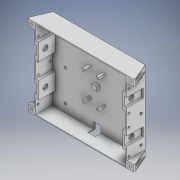
# Autodesk Inventor part: IPC Rear Panel v2
Saved by Autodesk Inventor 2022 (Build 260153000, 153)
## iProperties
Created: 2021-12-31
Part Number: IPC Rear Panel v2
Material: Generic
Document SubType Name: Modeling
Designer: solor
Density: 1 g/cm^3
Appearance: Default
Author: solor
Autodesk Inventor part; units mm, degrees
ref_plane "YZ Plane" through (0, 0, 0) normal (1, 0, 0) x (0, 1, 0)
ref_plane "XZ Plane" through (0, 0, 0) normal (0, 1, 0) x (-1, 0, 0)
sketch "Sketch1" plane through (0, 0, 0) normal (0, 0, 1) x (1, 0, 0)
  line L0 (0, 106) -> (0, 97)
  line L1 (0, 97) -> (9, 97)
  line L2 (9, 9) -> (0, 9)
  line L3 (0, 9) -> (0, 0)
  line L4 (138.8502, 0) -> (138.8502, 9)
  line L5 (138.8502, 9) -> (129.8502, 9)
  line L6 (129.8502, 97) -> (138.8502, 97)
  line L7 (138.8502, 97) -> (138.8502, 106)
  circle A0 centre (134.3502, 101.5) radius 1.65
  circle A1 centre (134.3502, 4.5) radius 1.65
  circle A2 centre (4.5, 4.5) radius 1.65
  circle A3 centre (4.5, 101.5) radius 1.65
  line L8 (9, 106) -> (9, 0)
  line L9 (129.8502, 0) -> (129.8502, 106)
  line L10 (0, 106) -> (9, 106)
  line L11 (9, 106) -> (129.8502, 106)
  line L12 (129.8502, 106) -> (138.8502, 106)
  line L13 (138.8502, 0) -> (129.8502, 0)
  line L14 (129.8502, 0) -> (9, 0)
  line L15 (9, 0) -> (0, 0)
  line L16 (10.3351, 1.335) -> (128.5151, 1.335)
  line L17 (128.5151, 1.335) -> (128.5151, 104.665)
  line L18 (128.5151, 104.665) -> (10.3351, 104.665)
  line L19 (10.3351, 104.665) -> (10.3351, 1.335)
  line L20 (10.3351, 1.335) -> (128.5151, 104.665) construction
  line L21 (128.5151, 1.335) -> (10.3351, 104.665) construction
  point P0 (0, 0)
  point P1 (69.4251, 53)
  dimension "d0" = 118.18
  dimension "d1" = 103.33
  constraints: 44 end point, 4 centre point, 4 collinear, 4 point on line, 3 parallel, 2 horizontal, 2 midpoint, 1 perpendicular
  measures "d0" distance of L18.end L17.end
  measures "d1" distance of L17.end L16.end
sketch "Sketch2" plane through (0, 0, 0) normal (0, 0, 1) x (1, 0, 0)
  line L0 (9, 46.5) -> (9, 9)
  line L1 (0, 46.5) -> (9, 46.5)
  line L2 (0, 59.5) -> (0, 46.5)
  line L3 (9, 59.5) -> (0, 59.5)
  line L4 (9, 88) -> (9, 59.5)
  line L5 (9, 97) -> (9, 88)
  line L6 (9, 97) -> (0, 97)
  line L7 (0, 97) -> (0, 106)
  line L8 (117.3502, 0) -> (3.5, 0)
  line L9 (117.3502, 0) -> (129.8502, 0)
  line L10 (138.8502, 106) -> (138.8502, 97)
  line L11 (138.8502, 97) -> (129.8502, 97)
  line L12 (129.8502, 88) -> (129.8502, 97)
  line L13 (129.8502, 59.5) -> (129.8502, 88)
  line L14 (138.8502, 59.5) -> (129.8502, 59.5)
  line L15 (138.8502, 46.5) -> (138.8502, 59.5)
  line L16 (129.8502, 46.5) -> (138.8502, 46.5)
  line L17 (129.8502, 9) -> (129.8502, 46.5)
  line L18 (129.8502, 9) -> (138.8502, 9)
  line L19 (138.8502, 9) -> (138.8502, 0)
  line L20 (138.8502, 0) -> (126.3502, 0)
  line L21 (12.5, 0) -> (126.3502, 0)
  line L22 (12.5, 0) -> (0, 0)
  line L23 (0, 0) -> (0, 9)
  line L24 (0, 9) -> (9, 9)
  circle A0 centre (4.5, 4.5) radius 1.65
  circle A1 centre (134.3502, 4.5) radius 1.65
  circle A2 centre (134.3502, 101.5) radius 1.65
  circle A3 centre (4.5, 101.5) radius 1.65
  constraints: 50 end point, 4 centre point
extrude "Extrusion1" add sketch "Sketch1" along normal blind 24 contours L11 L9 L14 L8
extrude "Extrusion2" add sketch "Sketch1" along normal blind 2.56 contours L19 L18 L17 L16
sketch "Sketch3" plane through (0, 0, 24) normal (0, 0, 1) x (1, 0, 0)
  line L0 (138.8502, 97) -> (129.8502, 97) projected
  line L1 (138.8502, 106) -> (138.8502, 97) projected
  line L2 (129.8502, 106) -> (138.8502, 106) projected
  circle A0 centre (134.3502, 101.5) radius 1.65 projected
  line L3 (129.8502, 0) -> (129.8502, 106) projected
  line L4 (129.8502, 9) -> (138.8502, 9) projected
  line L5 (138.8502, 9) -> (138.8502, 0) projected
  line L6 (138.8502, 0) -> (126.3502, 0) projected
  circle A1 centre (134.3502, 4.5) radius 1.65 projected
  line L7 (12.5, 0) -> (0, 0) projected
  line L8 (0, 0) -> (0, 9) projected
  line L9 (0, 9) -> (9, 9) projected
  circle A2 centre (4.5, 4.5) radius 1.65 projected
  line L10 (9, 97) -> (0, 97) projected
  line L11 (0, 97) -> (0, 106) projected
  line L12 (0, 106) -> (9, 106) projected
  circle A3 centre (4.5, 101.5) radius 1.65 projected
  line L13 (9, 106) -> (9, 0) projected
extrude "Extrusion3" add sketch "Sketch3" against normal blind 2.56
sketch "Sketch4" plane through (9, 0, 0) normal (0, -1, 0) x (1, 0, 0)
  line L0 (0, 21.44) -> (-9, 21.44) projected
  line L1 (0, 0) -> (0, 21.44) projected
  line L2 (-9, 21.44) -> (0, 0)
  line L3 (0, 0) -> (0, 21.44)
  line L4 (0, 21.44) -> (-9, 21.44)
  line L5 (120.8502, 0) -> (120.8502, 21.44) projected
  line L6 (129.8502, 21.44) -> (120.8502, 21.44) projected
  line L7 (120.8502, 21.44) -> (129.8502, 21.44)
  line L8 (129.8502, 21.44) -> (120.8502, 0)
  line L9 (120.8502, 0) -> (120.8502, 21.44)
  point P0 (-9, 0)
  constraints: 12 end point, 2 perpendicular, 1 collinear, 1 horizontal
extrude "Extrusion4" add sketch "Sketch4" against normal blind 106
sketch "Sketch5" plane through (138.8502, 97, 24) normal (1, 0, 0) x (0, 0, -1)
  line L0 (2.56, 0) -> (2.56, -88) projected
  line L1 (2.56, -88) -> (25.0861, -88)
  line L2 (24, -97) -> (24, 9) projected
  line L3 (25.0861, -88) -> (25.0861, 0)
  line L4 (25.0861, 0) -> (-1.4553, 0)
  line L5 (-1.4553, 0) -> (-1.4553, -88)
  line L6 (2.56, -88) -> (0, -88) projected
  line L7 (-1.4553, -88) -> (2.56, -88)
  line L8 (2.56, -97) -> (2.56, -88) projected
  line L9 (2.56, -88) -> (2.56, -89.3)
  line L10 (2.56, -89.3) -> (24, -89.3)
  line L11 (24, -89.3) -> (24, -95.7)
  line L12 (24, -95.7) -> (2.56, -95.7)
  line L13 (2.56, -95.7) -> (2.56, -89.3)
  line L14 (2.56, 9) -> (2.56, 0) projected
  line L15 (2.56, 0) -> (2.56, 1.3)
  line L16 (2.56, 1.3) -> (24, 1.3)
  line L17 (24, 1.3) -> (24, 7.7)
  line L18 (24, 7.7) -> (2.56, 7.7)
  line L19 (2.56, 7.7) -> (2.56, 1.3)
  point P0 (2.56, 7.7)
  point P1 (24, 0)
  point P2 (24, -88)
  dimension "d10" = 1.3
  dimension "d11" = 6.4
  dimension "d12" = 1.3
  dimension "d13" = 6.4
  constraints: 30 end point, 10 perpendicular, 9 point on line, 1 collinear
  measures "d10" distance of L0.end L9.end
  measures "d11" distance of L10.end L11.end
  measures "d12" distance of L0.start L15.end
  measures "d13" distance of L16.end L17.end
extrude "Extrusion5" cut sketch "Sketch5" against normal blind 9 contours L4 L2 L1 L0 | L14 L18 L2 L16 | L10 L2 L12 L8
sketch "Sketch6" plane through (0, 0, 24) normal (-1, 0, 0) x (0, 0, 1)
  line L0 (-24, 1.3) -> (-24, 7.7) projected
  line L1 (-2.56, 7.7) -> (-24, 7.7) projected
  line L2 (-2.56, 1.3) -> (-2.56, 7.7) projected
  line L3 (-24, 1.3) -> (-2.56, 1.3) projected
  line L4 (-24, 97) -> (0, 97) projected
  line L5 (0, 9) -> (0, 97) projected
  line L6 (0, 9) -> (-24, 9) projected
  line L7 (-24, 9) -> (-24, 97) projected
  line L8 (-2.56, 98.3) -> (-2.56, 104.7) projected
  line L9 (-24, 98.3) -> (-2.56, 98.3) projected
  line L10 (-24, 98.3) -> (-24, 104.7) projected
  line L11 (-2.56, 104.7) -> (-24, 104.7) projected
  point P0 (-24, 0)
extrude "Extrusion6" cut sketch "Sketch6" against normal blind 9
ref_plane "Work Plane1" through (0, 0, 37.6398) normal (0, 0, 1) x (1, 0, 0)
sketch "Sketch7" plane through (0, 0, 37.6398) normal (0, 0, 1) x (1, 0, 0)
  line L0 (0, 59.5) -> (0, 46.5) projected
  line L1 (9, 59.5) -> (0, 59.5) projected
  line L2 (0, 46.5) -> (9, 46.5) projected
  line L3 (9, 97) -> (9, 9) projected
  line L4 (138.8502, 46.5) -> (138.8502, 59.5) projected
  line L5 (129.8502, 46.5) -> (138.8502, 46.5) projected
  line L6 (138.8502, 59.5) -> (129.8502, 59.5) projected
  line L7 (129.8502, 9) -> (129.8502, 97) projected
  point P0 (0, 0)
sketch "Sketch8" plane through (9, 9, 24) normal (-1, 0, 0) x (0, 0, 1)
  line L0 (32.712, 88) -> (32.712, 50.5) construction
  line L1 (17.6212, 69.25) -> (-0.9488, 69.25) construction
  line L2 (0, -16.3005) -> (-7, -16.3005) construction
  line L3 (13.6398, 37.5) -> (13.6398, 50.5) construction
  line L4 (13.6398, 44) -> (-26.4859, 44) construction
  line L5 (-34.861, 44) -> (-34.861, 88) construction
  circle A0 centre (-7, 66) radius 21.6937
  circle A1 centre (-7, 66) radius 5.75
  point P0 (-24, -9)
  dimension "d21" = 18.57
  dimension "d23" = 7
  dimension "d24" = 11.5
  constraints: 10 end point, 3 horizontal, 2 centre point, 2 vertical, 1 coincident, 1 midpoint
  measures "d21" distance of L1.start L1.end
  measures "d23" distance of L2.start L2.end
  measures "d24" diameter of A1
sketch "Sketch9" plane through (0, 0, 24) normal (0, 0, 1) x (1, 0, 0)
  line L0 (14.2, 69.25) -> (14.2, 80.75)
  line L1 (14.2, 80.75) -> (9, 80.75)
  line L2 (9, 86.2) -> (16.78, 86.2)
  line L3 (16.78, 86.2) -> (16.78, 63.8)
  line L4 (16.78, 63.8) -> (9, 63.8)
  line L5 (9, 63.8) -> (9, 69.25)
  line L6 (9, 80.75) -> (9, 86.2)
  line L7 (9, 97) -> (9, 9) projected
  line L8 (9, 69.25) -> (14.2, 69.25)
  point P0 (0, 0)
  dimension "d29" = 7.78
  dimension "d30" = 22.4
  constraints: 16 end point, 2 perpendicular, 1 collinear, 1 parallel, 1 vertical
  measures "d29" distance of L2.start L2.end
  measures "d30" distance of L2.end L3.end
extrude "Extrusion8" add sketch "Sketch9" against normal blind 24 contours L0 L1 L6 L2 L3 L4 L5 L8
sketch "Sketch10" plane through (0, 0, 24) normal (0, 0, 1) x (1, 0, 0)
  line L0 (16.78, 63.8) -> (16.78, 86.2) projected
  line L1 (14.2, 69.25) -> (10.3351, 69.25) projected
  line L2 (14.2, 80.75) -> (14.2, 69.25) projected
  line L3 (10.3351, 69.25) -> (14.2, 69.25) projected
  line L4 (14.2, 69.25) -> (14.2, 80.75) projected
  line L5 (14.2, 80.75) -> (10.3351, 80.75) projected
  line L6 (10.3351, 69.25) -> (10.3351, 80.75) projected
  line L7 (10.3351, 104.665) -> (128.5151, 104.665) projected
  line L8 (69.4251, 104.665) -> (69.4251, 1.335)
  line L9 (128.5151, 1.335) -> (10.3351, 1.335) projected
  line L10 (9, 53) -> (129.7844, 53)
  line L11 (16.78, 86.2) -> (10.3351, 86.2) projected
  line L12 (10.3351, 69.25) -> (10.3351, 80.75) projected
  line L13 (10.3351, 80.75) -> (9, 80.75)
  line L14 (9, 80.75) -> (9, 69.25)
  line L15 (9, 69.25) -> (10.3351, 69.25)
  line L16 (10.3351, 80.75) -> (14.2, 80.75) projected
  line L17 (10.3351, 80.75) -> (10.3351, 69.25)
  line L18 (16.78, 63.8) -> (10.3351, 63.8) projected
  line L19 (10.3351, 63.8) -> (10.3351, 69.25)
  line L20 (10.3351, 86.2) -> (10.3351, 80.75)
  line L21 (122.0702, 63.8) -> (122.0702, 86.2)
  line L22 (124.6502, 69.25) -> (128.5151, 69.25)
  line L23 (124.6502, 80.75) -> (124.6502, 69.25)
  line L24 (128.5151, 69.25) -> (124.6502, 69.25)
  line L25 (124.6502, 69.25) -> (124.6502, 80.75)
  line L26 (124.6502, 80.75) -> (128.5151, 80.75)
  line L27 (128.5151, 69.25) -> (128.5151, 80.75)
  line L28 (122.0702, 86.2) -> (128.5151, 86.2)
  line L29 (128.5151, 69.25) -> (128.5151, 80.75)
  line L30 (128.5151, 80.75) -> (129.8502, 80.75)
  line L31 (129.8502, 80.75) -> (129.8502, 69.25)
  line L32 (129.8502, 69.25) -> (128.5151, 69.25)
  line L33 (128.5151, 80.75) -> (124.6502, 80.75)
  line L34 (128.5151, 80.75) -> (128.5151, 69.25)
  line L35 (122.0702, 63.8) -> (128.5151, 63.8)
  line L36 (128.5151, 63.8) -> (128.5151, 69.25)
  line L37 (128.5151, 86.2) -> (128.5151, 80.75)
  line L38 (16.78, 42.2) -> (16.78, 19.8)
  line L39 (14.2, 36.75) -> (10.3351, 36.75)
  line L40 (14.2, 25.25) -> (14.2, 36.75)
  line L41 (10.3351, 36.75) -> (14.2, 36.75)
  line L42 (14.2, 36.75) -> (14.2, 25.25)
  line L43 (14.2, 25.25) -> (10.3351, 25.25)
  line L44 (10.3351, 36.75) -> (10.3351, 25.25)
  line L45 (16.78, 19.8) -> (10.3351, 19.8)
  line L46 (10.3351, 36.75) -> (10.3351, 25.25)
  line L47 (10.3351, 25.25) -> (9, 25.25)
  line L48 (9, 25.25) -> (9, 36.75)
  line L49 (9, 36.75) -> (10.3351, 36.75)
  line L50 (10.3351, 25.25) -> (14.2, 25.25)
  line L51 (10.3351, 25.25) -> (10.3351, 36.75)
  line L52 (16.78, 42.2) -> (10.3351, 42.2)
  line L53 (10.3351, 42.2) -> (10.3351, 36.75)
  line L54 (10.3351, 19.8) -> (10.3351, 25.25)
  line L55 (122.0702, 42.2) -> (128.5151, 42.2)
  line L56 (124.6502, 36.75) -> (128.5151, 36.75)
  line L57 (128.5151, 36.75) -> (124.6502, 36.75)
  line L58 (128.5151, 42.2) -> (128.5151, 36.75)
  line L59 (129.8502, 36.75) -> (128.5151, 36.75)
  line L60 (124.6502, 25.25) -> (124.6502, 36.75)
  line L61 (124.6502, 36.75) -> (124.6502, 25.25)
  line L62 (122.0702, 42.2) -> (122.0702, 19.8)
  line L63 (128.5151, 25.25) -> (124.6502, 25.25)
  line L64 (128.5151, 36.75) -> (128.5151, 25.25)
  line L65 (128.5151, 25.25) -> (128.5151, 36.75)
  line L66 (128.5151, 36.75) -> (128.5151, 25.25)
  line L67 (124.6502, 25.25) -> (128.5151, 25.25)
  line L68 (122.0702, 19.8) -> (128.5151, 19.8)
  line L69 (129.8502, 25.25) -> (129.8502, 36.75)
  line L70 (128.5151, 19.8) -> (128.5151, 25.25)
  line L71 (128.5151, 25.25) -> (129.8502, 25.25)
  point P0 (0, 0)
  constraints: 118 end point, 39 symmetric about line, 3 perpendicular, 2 horizontal, 2 midpoint, 1 collinear
extrude "Extrusion9" cut sketch "Sketch10" against normal blind 21.44 contours L15 L14 L13 L6 | L27 L30 L31 L32 | L44 L47 L48 L49 | L59 L69 L71 L64
extrude "Extrusion10" add sketch "Sketch10" against normal blind 21.44 contours L21 L28 L37 L26 L23 L22 L36 L35 | L38 L45 L54 L43 L40 L39 L53 L52 | L55 L58 L56 L60 L63 L70 L68 L62
sketch "Sketch11" plane through (9, 9, 0) normal (-1, 0, 0) x (0, 0, 1)
  line L0 (2.56, 33.2) -> (2.56, 10.8) projected
  circle A0 centre (17, 66) radius 21.6937 projected
  line L1 (24, 27.75) -> (2.56, 27.75) projected
  circle A1 centre (17, 22) radius 21.6937
  circle A2 centre (17, 66) radius 3.525
  circle A3 centre (17, 22) radius 3.525
  line L2 (9.65, 22) -> (9.65, 23.5)
  line L3 (9.65, 23.5) -> (7.65, 23.5)
  line L4 (7.65, 23.5) -> (7.65, 20.5)
  line L5 (7.65, 20.5) -> (9.65, 20.5)
  line L6 (9.65, 20.5) -> (9.65, 22)
  line L7 (37.6398, 37.5) -> (37.6398, 50.5) projected
  line L8 (37.6398, 44) -> (44.1108, 44)
  line L9 (9.65, 66) -> (9.65, 64.5)
  line L10 (9.65, 64.5) -> (7.65, 64.5)
  line L11 (7.65, 64.5) -> (7.65, 67.5)
  line L12 (7.65, 67.5) -> (9.65, 67.5)
  line L13 (9.65, 67.5) -> (9.65, 66)
  line L14 (17, 31.5257) -> (17, 36.9305)
  line L15 (24.35, 22) -> (24.35, 23.5)
  line L16 (24.35, 23.5) -> (26.35, 23.5)
  line L17 (26.35, 23.5) -> (26.35, 20.5)
  line L18 (26.35, 20.5) -> (24.35, 20.5)
  line L19 (24.35, 20.5) -> (24.35, 22)
  line L20 (24.35, 64.5) -> (26.35, 64.5)
  line L21 (24.35, 66) -> (24.35, 64.5)
  line L22 (24.35, 67.5) -> (24.35, 66)
  line L23 (26.35, 64.5) -> (26.35, 67.5)
  line L24 (26.35, 67.5) -> (24.35, 67.5)
  point P0 (0, -9)
  point P1 (2.56, 22)
  dimension "d37" = 7.05
  dimension "d38" = 7.05
  constraints: 44 end point, 15 symmetric about line, 4 perpendicular, 4 point on line, 3 centre point, 2 coincident, 2 midpoint, 1 horizontal, 1 vertical
  measures "d37" diameter of A2
  measures "d38" diameter of A3
extrude "Extrusion11" cut sketch "Sketch11" against normal blind 146.835 contours A2 | A3 | L6 L5 L4 L3 L2 | L9 L10 L11 L12 L13
sketch "Sketch12" plane through (0, 0, 24) normal (0, -1, 0) x (1, 0, 0)
  line L0 (66.4498, -24.1403) -> (72.4005, -24.1403)
  line L1 (72.4005, -24.1403) -> (72.4005, -17.0714)
  line L2 (72.4005, -17.0714) -> (66.4498, -17.0714)
  line L3 (66.4498, -17.0714) -> (66.4498, -24.1403)
  line L4 (66.4498, -24.1403) -> (72.4005, -17.0714) construction
  line L5 (72.4005, -24.1403) -> (66.4498, -17.0714) construction
  point P0 (0, -24)
  point P1 (69.4251, -20.6058)
  constraints: 12 end point, 2 midpoint, 2 parallel, 1 horizontal, 1 perpendicular
extrude "Extrusion12" cut sketch "Sketch12" against normal blind 5.5475
sketch "Sketch13" plane through (0, 0, 2.56) normal (0, 0, 1) x (1, 0, 0)
  line L0 (66.4498, 1.335) -> (66.4498, 5.5475) projected
  line L1 (66.4498, 5.5475) -> (72.4005, 5.5475) projected
  line L2 (72.4005, 5.5475) -> (72.4005, 1.335) projected
  line L3 (128.5151, 1.335) -> (72.4005, 1.335) projected
  line L4 (128.5151, 19.8) -> (128.5151, 1.335) projected
  line L5 (128.5151, 19.8) -> (122.0702, 19.8) projected
  line L6 (122.0702, 19.8) -> (122.0702, 42.2) projected
  line L7 (122.0702, 42.2) -> (128.5151, 42.2) projected
  line L8 (128.5151, 63.8) -> (128.5151, 42.2) projected
  line L9 (128.5151, 63.8) -> (122.0702, 63.8) projected
  line L10 (122.0702, 63.8) -> (122.0702, 86.2) projected
  line L11 (122.0702, 86.2) -> (128.5151, 86.2) projected
  line L12 (128.5151, 104.665) -> (128.5151, 86.2) projected
  line L13 (10.3351, 104.665) -> (128.5151, 104.665) projected
  line L14 (10.3351, 86.2) -> (10.3351, 104.665) projected
  line L15 (10.3351, 86.2) -> (16.78, 86.2) projected
  line L16 (16.78, 86.2) -> (16.78, 63.8) projected
  line L17 (16.78, 63.8) -> (10.3351, 63.8) projected
  line L18 (10.3351, 42.2) -> (10.3351, 63.8) projected
  line L19 (10.3351, 42.2) -> (16.78, 42.2) projected
  line L20 (16.78, 42.2) -> (16.78, 19.8) projected
  line L21 (16.78, 19.8) -> (10.3351, 19.8) projected
  line L22 (10.3351, 1.335) -> (10.3351, 19.8) projected
  line L23 (66.4498, 1.335) -> (10.3351, 1.335) projected
  line L24 (61.1838, 36.7005) -> (78.4251, 70.8) construction
  line L25 (78.4251, 35.2) -> (60.4251, 70.8) construction
  line L26 (61.9251, 33.5865) -> (61.9251, 35.2)
  line L27 (69.4251, 57.7505) -> (69.4251, 50.8052)
  line L28 (66.4498, 53) -> (71.4698, 53)
  line L29 (61.9251, 72.4135) -> (61.9251, 70.8)
  line L30 (60.4251, 69.2995) -> (58.8116, 69.2995)
  line L31 (76.9251, 33.5865) -> (76.9251, 35.2)
  line L32 (78.4251, 36.7005) -> (80.0387, 36.7005)
  line L33 (76.9251, 72.4135) -> (76.9251, 70.8)
  line L34 (78.4251, 69.2995) -> (80.0387, 69.2995)
  line L35 (60.4251, 36.7005) -> (58.8116, 36.7005)
  line L36 (60.4251, 70.8) -> (60.4251, 69.2995)
  line L37 (60.4251, 36.7005) -> (60.4251, 35.2)
  line L38 (58.8116, 33.5865) -> (58.8116, 36.7005)
  line L39 (58.8116, 69.2995) -> (58.8116, 72.4135)
  line L40 (58.8116, 72.4135) -> (61.9251, 72.4135)
  line L41 (76.9251, 72.4135) -> (80.0387, 72.4135)
  line L42 (78.4251, 70.8) -> (76.9251, 70.8)
  line L43 (61.9251, 70.8) -> (60.4251, 70.8)
  line L44 (78.4251, 35.2) -> (78.4251, 36.7005)
  line L45 (78.4251, 69.2995) -> (78.4251, 70.8)
  line L46 (80.0387, 72.4135) -> (80.0387, 69.2995)
  line L47 (80.0387, 36.7005) -> (80.0387, 33.5865)
  line L48 (60.4251, 35.2) -> (61.9251, 35.2)
  line L49 (76.9251, 35.2) -> (78.4251, 35.2)
  line L50 (80.0387, 33.5865) -> (76.9251, 33.5865)
  line L51 (61.9251, 33.5865) -> (58.8116, 33.5865)
  line L52 (66.0452, 50.056) -> (72.805, 50.056)
  line L53 (72.805, 50.056) -> (72.805, 55.944)
  line L54 (72.805, 55.944) -> (66.0452, 55.944)
  line L55 (66.0452, 55.944) -> (66.0452, 50.056)
  line L56 (66.0452, 50.056) -> (72.805, 55.944) construction
  line L57 (72.805, 50.056) -> (66.0452, 55.944) construction
  point P0 (0, 0)
  point P1 (69.4251, 53)
  point P2 (61.9251, 32.5085)
  point P3 (57.4575, 36.7005)
  point P4 (61.9251, 73.4915)
  point P5 (61.9251, 69.2995)
  point P6 (57.4575, 69.2995)
  point P7 (76.9251, 32.5085)
  point P8 (81.3927, 36.7005)
  point P9 (76.9251, 73.4915)
  point P10 (76.9251, 69.2995)
  point P11 (81.3927, 69.2995)
  dimension "d47" = 18
  dimension "d48" = 35.6
  constraints: 68 end point, 18 parallel, 13 perpendicular, 7 symmetric about line, 4 horizontal, 3 midpoint, 1 point on line, 1 vertical
  measures "d47" distance of L25.end L24.end
  measures "d48" distance of L24.end L25.start
extrude "Extrusion13" add sketch "Sketch13" along normal blind 8.7225 contours L51 L38 L35 L37 L48 L26 | L29 L43 L36 L30 L39 L40 | L31 L49 L44 L32 L47 L50 | L41 L46 L34 L45 L42 L33
extrude "Extrusion14" add sketch "Sketch13" along normal blind 4 contours L55 L54 L53 L52
sketch "Sketch14" plane through (0, 0, 2.56) normal (0, 0, 1) x (1, 0, 0)
  line L0 (66.0452, 55.944) -> (66.0452, 50.056) projected
  line L1 (66.0452, 50.056) -> (72.805, 50.056) projected
  line L2 (72.805, 50.056) -> (72.805, 55.944) projected
  line L3 (72.805, 55.944) -> (66.0452, 55.944) projected
  line L4 (66.0452, 55.944) -> (72.805, 55.944) projected
  line L5 (72.805, 55.944) -> (72.805, 50.056) projected
  line L6 (72.805, 50.056) -> (66.0452, 50.056) projected
  line L7 (66.0452, 50.056) -> (66.0452, 55.944) projected
  line L8 (78.4251, 69.2995) -> (78.4251, 70.8) projected
  line L9 (78.4251, 70.8) -> (76.9251, 70.8) projected
  line L10 (76.9251, 70.8) -> (76.9251, 72.4135) projected
  line L11 (76.9251, 72.4135) -> (80.0387, 72.4135) projected
  line L12 (80.0387, 72.4135) -> (80.0387, 69.2995) projected
  line L13 (80.0387, 69.2995) -> (78.4251, 69.2995) projected
  line L14 (80.0387, 33.5865) -> (76.9251, 33.5865) projected
  line L15 (76.9251, 33.5865) -> (76.9251, 35.2) projected
  line L16 (76.9251, 35.2) -> (78.4251, 35.2) projected
  line L17 (78.4251, 35.2) -> (78.4251, 36.7005) projected
  line L18 (78.4251, 36.7005) -> (80.0387, 36.7005) projected
  line L19 (80.0387, 36.7005) -> (80.0387, 33.5865) projected
  line L20 (58.8116, 72.4135) -> (61.9251, 72.4135) projected
  line L21 (61.9251, 72.4135) -> (61.9251, 70.8) projected
  line L22 (61.9251, 70.8) -> (60.4251, 70.8) projected
  line L23 (60.4251, 70.8) -> (60.4251, 69.2995) projected
  line L24 (60.4251, 69.2995) -> (58.8116, 69.2995) projected
  line L25 (58.8116, 69.2995) -> (58.8116, 72.4135) projected
  line L26 (61.9251, 33.5865) -> (58.8116, 33.5865) projected
  line L27 (58.8116, 33.5865) -> (58.8116, 36.7005) projected
  line L28 (58.8116, 36.7005) -> (60.4251, 36.7005) projected
  line L29 (60.4251, 36.7005) -> (60.4251, 35.2) projected
  line L30 (60.4251, 35.2) -> (61.9251, 35.2) projected
  line L31 (61.9251, 35.2) -> (61.9251, 33.5865) projected
  line L32 (66.4498, 1.335) -> (66.4498, 5.5475) projected
  line L33 (66.4498, 5.5475) -> (72.4005, 5.5475) projected
  line L34 (72.4005, 5.5475) -> (72.4005, 1.335) projected
  line L35 (128.5151, 1.335) -> (72.4005, 1.335) projected
  line L36 (128.5151, 19.8) -> (128.5151, 1.335) projected
  line L37 (128.5151, 19.8) -> (122.0702, 19.8) projected
  line L38 (122.0702, 19.8) -> (122.0702, 42.2) projected
  line L39 (122.0702, 42.2) -> (128.5151, 42.2) projected
  line L40 (128.5151, 63.8) -> (128.5151, 42.2) projected
  line L41 (128.5151, 63.8) -> (122.0702, 63.8) projected
  line L42 (122.0702, 63.8) -> (122.0702, 86.2) projected
  line L43 (122.0702, 86.2) -> (128.5151, 86.2) projected
  line L44 (128.5151, 104.665) -> (128.5151, 86.2) projected
  line L45 (10.3351, 104.665) -> (128.5151, 104.665) projected
  line L46 (10.3351, 86.2) -> (10.3351, 104.665) projected
  line L47 (10.3351, 86.2) -> (16.78, 86.2) projected
  line L48 (16.78, 86.2) -> (16.78, 63.8) projected
  line L49 (16.78, 63.8) -> (10.3351, 63.8) projected
  line L50 (10.3351, 42.2) -> (10.3351, 63.8) projected
  line L51 (10.3351, 42.2) -> (16.78, 42.2) projected
  line L52 (16.78, 42.2) -> (16.78, 19.8) projected
  line L53 (16.78, 19.8) -> (10.3351, 19.8) projected
  line L54 (10.3351, 1.335) -> (10.3351, 19.8) projected
  line L55 (66.4498, 1.335) -> (10.3351, 1.335) projected
  line L56 (27.683, 93.762) -> (111.1672, 93.762)
  line L57 (111.1672, 93.762) -> (111.1672, 53.103)
  line L58 (111.1672, 53.103) -> (111.1672, 12.238)
  line L59 (111.1672, 12.238) -> (83.3035, 12.238)
  line L60 (83.3035, 12.238) -> (83.3035, 16.4505)
  line L61 (83.3035, 16.4505) -> (55.5468, 16.4505)
  line L62 (55.5468, 16.4505) -> (55.5468, 12.238)
  line L63 (55.5468, 12.238) -> (27.683, 12.238)
  line L64 (27.683, 12.238) -> (27.683, 52.897)
  line L65 (27.683, 52.897) -> (27.683, 93.762)
  circle A0 centre (27.683, 12.238) radius 1.65
  circle A1 centre (27.683, 52.897) radius 1.65
  circle A2 centre (27.683, 93.762) radius 1.65
  circle A3 centre (69.4251, 93.762) radius 1.65
  circle A4 centre (111.1672, 93.762) radius 1.65
  circle A5 centre (111.1672, 53.103) radius 1.65
  circle A6 centre (111.1672, 12.238) radius 1.65
  circle A7 centre (69.4251, 12.238) radius 1.65
  point P0 (0, 0)
  dimension "d55" = 3.3
  dimension "d56" = 3.3
  constraints: 20 end point, 8 centre point, 6 coincident, 1 midpoint, 9 other
  measures "d55" diameter of A0
  measures "d56" diameter of A1
extrude "Extrusion15" cut sketch "Sketch14" against normal blind 3.3 contours L65 A2 L56 | L56 A2 L65 | A3 L56 | L56 A3 | A1 L64 L65 | L65 L64 A1 | A4 L57 L56 | L56 L57 A4 | A0 L63 L64 | L64 L63 A0 | A5 L58 L57 | L57 L58 A5 | A6 L59 L58 | L58 L59 A6
sketch "Sketch15" plane through (129.8502, 9, 0) normal (1, 0, 0) x (0, 0, -1)
  line L0 (-24, 10.8) -> (-2.56, 10.8) projected
  line L1 (-24, 33.2) -> (-2.56, 33.2) projected
  line L2 (-24, 54.8) -> (-2.56, 54.8) projected
  line L3 (-24, 77.2) -> (-2.56, 77.2) projected
  line L4 (-24, 10.8) -> (-2.56, 10.8)
  line L5 (-2.56, 10.8) -> (-2.56, 0)
  line L6 (-2.56, -7.665) -> (-2.56, 10.8) projected
  line L7 (-21.44, -1.3) -> (0, -1.3) projected
  line L8 (-24, -9) -> (-24, 0) projected
  line L9 (-24, 0) -> (-2.56, 0)
  line L10 (0, 0) -> (-21.44, 0) projected
  line L11 (-24, 0) -> (-21.44, 0) projected
  line L12 (-24, 0) -> (-24, 10.8)
  line L13 (-21.2, 8) -> (-5.36, 8)
  line L14 (-5.36, 8) -> (-5.36, 2.8)
  line L15 (-5.36, 2.8) -> (-21.2, 2.8)
  line L16 (-21.2, 2.8) -> (-21.2, 8)
  circle A0 centre (-21.2, 2.8) radius 1.65
  circle A1 centre (-5.36, 8) radius 1.65
  line L17 (-24, 10.8) -> (-2.56, 10.8)
  line L18 (-2.56, 10.8) -> (-2.56, 0)
  line L19 (-24, 0) -> (-2.56, 0)
  line L20 (-24, 0) -> (-24, 10.8)
  line L21 (-21.2, 8) -> (-5.36, 8)
  line L22 (-5.36, 8) -> (-5.36, 2.8)
  line L23 (-5.36, 2.8) -> (-21.2, 2.8)
  line L24 (-21.2, 2.8) -> (-21.2, 8)
  circle A2 centre (-21.2, 2.8) radius 1.65
  circle A3 centre (-5.36, 8) radius 1.65
  line L25 (-24, 88) -> (-2.56, 88)
  line L26 (-2.56, 88) -> (-2.56, 77.2)
  line L27 (-24, 77.2) -> (-2.56, 77.2)
  line L28 (-24, 77.2) -> (-24, 88)
  line L29 (-21.2, 85.2) -> (-5.36, 85.2)
  line L30 (-5.36, 85.2) -> (-5.36, 80)
  line L31 (-5.36, 80) -> (-21.2, 80)
  line L32 (-21.2, 80) -> (-21.2, 85.2)
  circle A4 centre (-21.2, 80) radius 1.65
  circle A5 centre (-5.36, 85.2) radius 1.65
  line L33 (-2.56, 54.8) -> (-2.56, 77.2) projected
  line L34 (-2.56, 54.8) -> (-2.56, 33.2)
  line L35 (-2.56, 33.2) -> (-24, 33.2)
  line L36 (-24, 54.8) -> (-2.56, 54.8) projected
  line L37 (-24, 33.2) -> (-24, 54.8)
  line L38 (-24, 54.8) -> (-2.56, 54.8)
  line L39 (-21.2, 52) -> (-21.2, 36)
  line L40 (-21.2, 36) -> (-5.36, 36)
  line L41 (-5.36, 36) -> (-5.36, 52)
  line L42 (-5.36, 52) -> (-21.2, 52)
  circle A6 centre (-5.36, 44) radius 1.65
  circle A7 centre (-21.2, 36) radius 1.65
  circle A8 centre (-21.2, 52) radius 1.65
  point P0 (0, -9)
  dimension "d59" = 2.8
  dimension "d60" = 3.3
  dimension "d61" = 3.3
  dimension "d62" = 2.8
  dimension "d63" = 3.3
  dimension "d64" = 3.3
  dimension "d65" = 2.8
  dimension "d66" = 3.3
  dimension "d67" = 3.3
  dimension "d68" = 2.8
  constraints: 64 end point, 10 perpendicular, 9 centre point, 8 coincident, 1 collinear, 1 midpoint, 1 point on line, 1 vertical, 12 other
  measures "d59" distance between parallel lines of L12 L16
  measures "d60" diameter of A0
  measures "d61" diameter of A1
  measures "d62" distance between parallel lines of L20 L24
  measures "d63" diameter of A2
  measures "d64" diameter of A3
  measures "d65" distance between parallel lines of L28 L32
  measures "d66" diameter of A4
  measures "d67" diameter of A5
  measures "d68" distance between parallel lines of L37 L39
extrude "Extrusion16" cut sketch "Sketch15" against normal blind 139.825 contours A1 L14 L13 | L13 L14 A1 | A0 L15 L16 | L16 L15 A0 | A5 L30 L29 | L29 L30 A5 | A4 L31 L32 | L32 L31 A4 | L42 A8 L39 | L39 A8 L42 | A7 L40 L39 | L39 L40 A7 | A6 L41 | L41 A6
sketch "Sketch16" plane through (0, 0, 6.56) normal (0, 0, 1) x (1, 0, 0)
  line L0 (72.805, 55.944) -> (66.0452, 55.944) projected
  circle A0 centre (111.1672, 93.762) radius 1.65 projected
  circle A1 centre (27.683, 52.897) radius 1.65 projected
  circle A2 centre (111.1672, 53.103) radius 1.65 projected
  circle A3 centre (69.4251, 93.762) radius 1.65 projected
  circle A4 centre (27.683, 12.238) radius 1.65 projected
  circle A5 centre (111.1672, 12.238) radius 1.65 projected
  circle A6 centre (27.683, 93.762) radius 1.65 projected
  line L1 (66.0452, 55.944) -> (72.805, 55.944) projected
  line L2 (72.805, 55.944) -> (72.805, 50.056) projected
  line L3 (72.805, 50.056) -> (66.0452, 50.056) projected
  line L4 (66.0452, 50.056) -> (66.0452, 55.944) projected
  line L5 (78.4251, 69.2995) -> (78.4251, 70.8) projected
  line L6 (78.4251, 70.8) -> (76.9251, 70.8) projected
  line L7 (76.9251, 70.8) -> (76.9251, 72.4135) projected
  line L8 (76.9251, 72.4135) -> (80.0387, 72.4135) projected
  line L9 (80.0387, 72.4135) -> (80.0387, 69.2995) projected
  line L10 (80.0387, 69.2995) -> (78.4251, 69.2995) projected
  line L11 (80.0387, 33.5865) -> (76.9251, 33.5865) projected
  line L12 (76.9251, 33.5865) -> (76.9251, 35.2) projected
  line L13 (76.9251, 35.2) -> (78.4251, 35.2) projected
  line L14 (78.4251, 35.2) -> (78.4251, 36.7005) projected
  line L15 (78.4251, 36.7005) -> (80.0387, 36.7005) projected
  line L16 (80.0387, 36.7005) -> (80.0387, 33.5865) projected
  line L17 (58.8116, 72.4135) -> (61.9251, 72.4135) projected
  line L18 (61.9251, 72.4135) -> (61.9251, 70.8) projected
  line L19 (61.9251, 70.8) -> (60.4251, 70.8) projected
  line L20 (60.4251, 70.8) -> (60.4251, 69.2995) projected
  line L21 (60.4251, 69.2995) -> (58.8116, 69.2995) projected
  line L22 (58.8116, 69.2995) -> (58.8116, 72.4135) projected
  line L23 (61.9251, 33.5865) -> (58.8116, 33.5865) projected
  line L24 (58.8116, 33.5865) -> (58.8116, 36.7005) projected
  line L25 (58.8116, 36.7005) -> (60.4251, 36.7005) projected
  line L26 (60.4251, 36.7005) -> (60.4251, 35.2) projected
  line L27 (60.4251, 35.2) -> (61.9251, 35.2) projected
  line L28 (61.9251, 35.2) -> (61.9251, 33.5865) projected
  line L29 (66.4498, 1.335) -> (66.4498, 5.5475) projected
  line L30 (66.4498, 5.5475) -> (72.4005, 5.5475) projected
  line L31 (72.4005, 5.5475) -> (72.4005, 1.335) projected
  line L32 (128.5151, 1.335) -> (72.4005, 1.335) projected
  line L33 (128.5151, 19.8) -> (128.5151, 1.335) projected
  line L34 (128.5151, 19.8) -> (122.0702, 19.8) projected
  line L35 (122.0702, 19.8) -> (122.0702, 42.2) projected
  line L36 (122.0702, 42.2) -> (128.5151, 42.2) projected
  line L37 (128.5151, 63.8) -> (128.5151, 42.2) projected
  line L38 (128.5151, 63.8) -> (122.0702, 63.8) projected
  line L39 (122.0702, 63.8) -> (122.0702, 86.2) projected
  line L40 (122.0702, 86.2) -> (128.5151, 86.2) projected
  line L41 (128.5151, 104.665) -> (128.5151, 86.2) projected
  line L42 (10.3351, 104.665) -> (128.5151, 104.665) projected
  line L43 (10.3351, 86.2) -> (10.3351, 104.665) projected
  line L44 (10.3351, 86.2) -> (16.78, 86.2) projected
  line L45 (16.78, 86.2) -> (16.78, 63.8) projected
  line L46 (16.78, 63.8) -> (10.3351, 63.8) projected
  line L47 (10.3351, 42.2) -> (10.3351, 63.8) projected
  line L48 (10.3351, 42.2) -> (16.78, 42.2) projected
  line L49 (16.78, 42.2) -> (16.78, 19.8) projected
  line L50 (16.78, 19.8) -> (10.3351, 19.8) projected
  line L51 (10.3351, 1.335) -> (10.3351, 19.8) projected
  line L52 (66.4498, 1.335) -> (10.3351, 1.335) projected
  point P0 (0, 0)
extrude "Extrusion17" add sketch "Sketch16" against normal blind 4.6375 contours L2 L3 L4 L0
sketch "Sketch17" plane through (0, 0, 24) normal (0, -1, 0) x (1, 0, 0)
  line L0 (66.4498, -17.0714) -> (72.4005, -17.0714) projected
  line L1 (129.8502, -24) -> (9, -24) projected
  line L2 (66.4498, -24) -> (76.2098, -24) construction
  line L3 (69.4251, -14) -> (74.3001, -14)
  line L4 (74.3001, -14) -> (74.3001, -24)
  line L5 (69.4251, -14) -> (64.5501, -14)
  line L6 (64.5501, -14) -> (64.5501, -24)
  line L7 (64.5501, -24) -> (74.3001, -24)
  point P0 (0, -24)
  point P1 (69.4251, -17.0714)
  dimension "d79" = 4.875
  dimension "d80" = 4.875
  constraints: 12 end point, 4 point on line, 2 perpendicular, 1 collinear, 1 horizontal, 1 midpoint
  measures "d79" distance of L3.start L3.end
  measures "d80" distance of L3.start L5.end
extrude "Extrusion18" cut sketch "Sketch17" against normal blind 10
sketch "Sketch18" plane through (0, 0, 24) normal (0, 0, 1) x (1, 0, 0)
  line L0 (14.12, 31) -> (14.12, 36.75)
  line L1 (14.12, 36.75) -> (11.6, 36.75)
  line L2 (11.6, 36.75) -> (11.6, 25.25)
  line L3 (11.6, 25.25) -> (14.12, 25.25)
  line L4 (14.12, 25.25) -> (14.12, 31)
  line L5 (10.3351, 42.2) -> (10.3351, 63.8) projected
  line L6 (128.5151, 51.35) -> (128.5151, 54.65) projected
  line L7 (10.3351, 104.665) -> (128.5151, 104.665) projected
  line L8 (69.4251, 104.665) -> (69.4251, 1.335)
  line L9 (74.3001, 1.335) -> (64.5501, 1.335) projected
  line L10 (14.12, 75) -> (14.12, 69.25)
  line L11 (14.12, 69.25) -> (11.6, 69.25)
  line L12 (11.6, 69.25) -> (11.6, 80.75)
  line L13 (11.6, 80.75) -> (14.12, 80.75)
  line L14 (14.12, 80.75) -> (14.12, 75)
  line L15 (124.7302, 31) -> (124.7302, 36.75)
  line L16 (124.7302, 36.75) -> (127.2502, 36.75)
  line L17 (127.2502, 36.75) -> (127.2502, 25.25)
  line L18 (127.2502, 25.25) -> (124.7302, 25.25)
  line L19 (124.7302, 25.25) -> (124.7302, 31)
  line L20 (124.7302, 75) -> (124.7302, 69.25)
  line L21 (124.7302, 69.25) -> (127.2502, 69.25)
  line L22 (127.2502, 69.25) -> (127.2502, 80.75)
  line L23 (127.2502, 80.75) -> (124.7302, 80.75)
  line L24 (124.7302, 80.75) -> (124.7302, 75)
  point P0 (0, 0)
  constraints: 42 end point, 10 symmetric about line, 4 point on line, 2 midpoint, 2 perpendicular
extrude "Extrusion19" add sketch "Sketch18" against normal blind 21.75
sketch "Sketch19" plane through (122.0702, 63.8, 24) normal (-1, 0, 0) x (0, 0, 1)
  circle A0 centre (-7, 11.2) radius 3.525 projected
  circle A1 centre (-7, -32.8) radius 3.525 projected
  point P0 (-24, -63.8)
sketch "Sketch20" plane through (0, 0, 24) normal (0, 0, 1) x (1, 0, 0)
  line L0 (14.12, 36.75) -> (14.12, 25.25) projected
  line L1 (14.12, 36.75) -> (14.12, 42.5862)
  line L2 (14.12, 42.5862) -> (19.5196, 42.5862)
  line L3 (19.5196, 42.5862) -> (19.5196, 17.6797)
  line L4 (19.5196, 17.6797) -> (14.12, 17.6797)
  line L5 (14.12, 36.75) -> (14.12, 17.6797)
  line L6 (10.3351, 42.2) -> (10.3351, 63.8) projected
  line L7 (14.12, 69.25) -> (14.12, 80.75)
  line L8 (14.12, 69.25) -> (14.12, 63.4138)
  line L9 (14.12, 63.4138) -> (19.5196, 63.4138)
  line L10 (19.5196, 63.4138) -> (19.5196, 88.3203)
  line L11 (19.5196, 88.3203) -> (14.12, 88.3203)
  line L12 (14.12, 69.25) -> (14.12, 88.3203)
  line L13 (10.3351, 104.665) -> (128.5151, 104.665) projected
  line L14 (69.4251, 104.665) -> (69.4251, 8.5462)
  line L15 (74.3001, 10) -> (64.5501, 10) projected
  line L16 (124.7302, 36.75) -> (124.7302, 25.25)
  line L17 (124.7302, 36.75) -> (124.7302, 42.5862)
  line L18 (124.7302, 42.5862) -> (119.3306, 42.5862)
  line L19 (119.3306, 42.5862) -> (119.3306, 17.6797)
  line L20 (119.3306, 17.6797) -> (124.7302, 17.6797)
  line L21 (124.7302, 36.75) -> (124.7302, 17.6797)
  line L22 (124.7302, 69.25) -> (124.7302, 80.75)
  line L23 (124.7302, 69.25) -> (124.7302, 63.4138)
  line L24 (124.7302, 63.4138) -> (119.3306, 63.4138)
  line L25 (119.3306, 63.4138) -> (119.3306, 88.3203)
  line L26 (119.3306, 88.3203) -> (124.7302, 88.3203)
  line L27 (124.7302, 69.25) -> (124.7302, 88.3203)
  point P0 (0, 0)
  constraints: 48 end point, 12 symmetric about line, 4 perpendicular, 4 point on line, 1 collinear, 1 midpoint
extrude "Extrusion21" cut sketch "Sketch20" against normal blind 21.44
sketch "Sketch21" plane through (11.6, 69.25, 24) normal (-1, 0, 0) x (0, 0, 1)
  circle A0 centre (-7, 5.75) radius 3.525 projected
  line L0 (-7, 5.75) -> (-8.5, 5.75) construction
  circle A1 centre (-8.5, 5.75) radius 3.525
  circle A2 centre (-8.5, -38.7569) radius 3.525
  point P0 (-24, -69.25)
  dimension "d91" = 1.5
  constraints: 2 centre point, 2 end point, 1 coincident, 1 horizontal
  measures "d91" distance of L0.start L0.end
extrude "Extrusion22" cut sketch "Sketch21" along normal mid plane 759.6275 contours A1 A0 | A0 A1 | A2 picked at (-8.6572, 5.75) picked at (-10.9988, 5.8895)
sketch "Sketch23" plane through (0, 0, 0) normal (0, 0, -1) x (-1, 0, 0)
  line L0 (-74.3001, 0) -> (-74.3001, 10) projected
  line L1 (-74.3001, 10) -> (-64.5501, 10) projected
  line L2 (-64.5501, 10) -> (-64.5501, 0) projected
  line L3 (-9, 0) -> (-64.5501, 0) projected
  line L4 (-9, 1.3) -> (-9, 0) projected
  line L5 (-9, 7.7) -> (-9, 1.3) projected
  line L6 (-9, 9) -> (-9, 7.7) projected
  line L7 (-9, 97) -> (-9, 9) projected
  line L8 (-9, 98.3) -> (-9, 97) projected
  line L9 (-9, 104.7) -> (-9, 98.3) projected
  line L10 (-9, 106) -> (-9, 104.7) projected
  line L11 (-129.8502, 106) -> (-9, 106) projected
  line L12 (-129.8502, 104.7) -> (-129.8502, 106) projected
  line L13 (-129.8502, 98.3) -> (-129.8502, 104.7) projected
  line L14 (-129.8502, 97) -> (-129.8502, 98.3) projected
  line L15 (-129.8502, 9) -> (-129.8502, 97) projected
  line L16 (-129.8502, 7.7) -> (-129.8502, 9) projected
  line L17 (-129.8502, 1.3) -> (-129.8502, 7.7) projected
  line L18 (-129.8502, 0) -> (-129.8502, 1.3) projected
  line L19 (-74.3001, 0) -> (-129.8502, 0) projected
  circle A0 centre (-27.683, 93.762) radius 1.65 projected
  circle A1 centre (-111.1672, 12.238) radius 1.65 projected
  circle A2 centre (-27.683, 12.238) radius 1.65 projected
  circle A3 centre (-69.4251, 93.762) radius 1.65 projected
  circle A4 centre (-111.1672, 53.103) radius 1.65 projected
  circle A5 centre (-27.683, 52.897) radius 1.65 projected
  circle A6 centre (-111.1672, 93.762) radius 1.65 projected
  point P0 (0, 0)
  dimension "d94" = 41.7421
  dimension "d95" = 12.238
  dimension "d96" = 52.897
  dimension "d97" = 93.762
  measures "d94" distance of A3.centre A6.centre
  measures "d95" distance from line of L11 A6.centre
  measures "d96" distance from line of A4.centre L11
  measures "d97" distance from line of A1.centre L11
equation "\"d57\" = d56"
body "Solid1"
